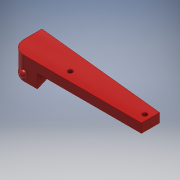
# Autodesk Inventor part: ArmExtension
Saved by Autodesk Inventor 2018.3 (Build 223284000, 284)
## iProperties
Created: 2020-03-24
Part Number: ArmExtension
Material: Generic
Document SubType Name: Modeling
Designer: Ivan
Density: 1 g/cm^3
Appearance: Default
Author: Ivan
Autodesk Inventor part; units mm, degrees
ref_plane "YZ Plane" through (0, 0, 0) normal (1, 0, 0) x (0, 1, 0)
ref_plane "XZ Plane" through (0, 0, 0) normal (0, 1, 0) x (-1, 0, 0)
ref_plane "XY Plane" through (0, 0, 0) normal (0, 0, 1) x (1, 0, 0)
sketch "Sketch1" plane through (0, 0, 0) normal (0, 0, 1) x (1, 0, 0)
  line L0 (-58, 14) -> (0, 14)
  line L1 (0, 14) -> (0, 0)
  line L2 (0, 0) -> (-58, 0)
  line L3 (-58, 0) -> (-58, 14)
  line L4 (-69.6, 0) -> (11.6, 0) projected
  point P0 (0, 0)
  dimension "d0" = 58
  dimension "d1" = 14
  constraints: 8 end point, 2 parallel, 1 collinear, 1 horizontal, 1 perpendicular
  measures "d0" distance of L0.start L0.end
  measures "d1" distance of L0.end L1.end
extrude "Extrusion1" add sketch "Sketch1" along normal blind 4
sketch "Sketch2" plane through (0, 0, 4) normal (0, 0, 1) x (1, 0, 0)
  circle A0 centre (-2.5, 4) radius 1
  line L0 (0, 0) -> (0, 14) projected
  circle A1 centre (-35.5, 4) radius 1
  line L1 (-58, 0) -> (0, 0) projected
  dimension "d4" = 2
  dimension "d6" = 2
  dimension "d7" = 33
  dimension "d22" = 4
  constraints: 2 centre point, 1 horizontal alignment
  measures "d4" diameter of A0
  measures "d6" diameter of A1
  measures "d7" distance of A0.centre A1.centre
  measures "d22" distance from line of L1 A0.centre
extrude "Extrusion2" cut sketch "Sketch2" against normal through all
sketch "Sketch3" plane through (-58, 0, 0) normal (-1, 0, 0) x (0, 0, 1)
  line L0 (0, 0) -> (0, 14) projected
  line L1 (0, 0) -> (4, 0) projected
  line L2 (0, 14) -> (0, 0)
  line L3 (0, 0) -> (-6, 0)
  line L4 (-6, 0) -> (0, 14)
  dimension "d10" = 6
  constraints: 6 end point, 2 perpendicular
  measures "d10" distance of L0.start L3.end
extrude "Extrusion3" add sketch "Sketch3" against normal blind 12
ref_plane "Work Plane1" through (-52, 0, 4) normal (-1, 0, 0) x (0, 0, 1)
fillet "Fillet1" radius 6 1 edges at (-58, 0, -1)
chamfer "Chamfer1" distance 6 distance2 58 1 edges at (0, 14, 2) measured on face at (0, 13.5, 2)
sketch "Sketch5" plane through (-52, 0, 4) normal (-1, 0, 0) x (0, 0, 1)
  arc A0 (-7, -1.5) -> (-8.5, 0) centre (-7, 0) ccw
  line L0 (-7, 0) -> (-7, 1.5)
  line L1 (-7, -1.5) -> (-7, 0)
  line L2 (-7, 0) -> (-5.5, 0)
  point P0 (-10, 0)
  dimension "d26" = 3
  dimension "d27" = 3
  constraints: 6 end point, 4 point on circle, 1 centre point, 1 collinear, 1 horizontal alignment, 1 point on line
  measures "d26" diameter of A0
  measures "d27" distance of point (-10, 0) L0.start
revolve "Revolution2" add sketch "Sketch5" angle 360 about axis through (-52, -1.5, -3) along (0, 1, 0)
body "Solid1"
